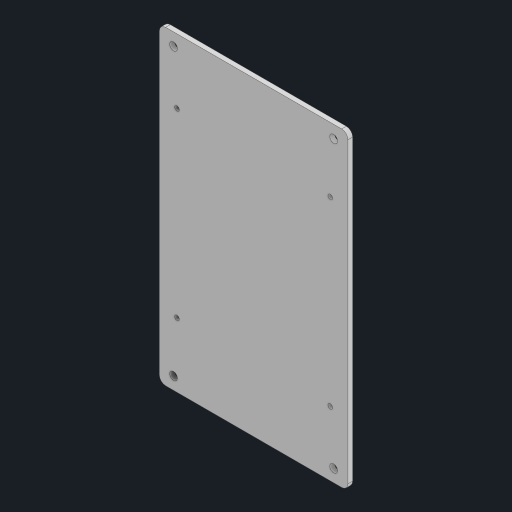
# Autodesk Inventor part: TauControllerCover
Saved by Autodesk Inventor 2023 (Build 270158000, 158)
## iProperties
Created: 2023-07-03
Part Number: TauControllerCover
Material: Generic
Document SubType Name: Sheet Metal
Designer: valer
Density: 1 g/cm^3
Sheet Metal Rule: Default
Appearance: Default
Author: valer
Autodesk Inventor part; units mm, degrees
ref_plane "YZ Plane" through (0, 0, 0) normal (1, 0, 0) x (0, 1, 0)
ref_plane "XZ Plane" through (0, 0, 0) normal (0, 1, 0) x (-1, 0, 0)
ref_plane "XY Plane" through (0, 0, 0) normal (0, 0, 1) x (1, 0, 0)
sketch "Sketch1" plane through (0, 0, 0) normal (0, 0, 1) x (1, 0, 0)
  line L0 (-28.15, 49.6305) -> (28.15, 49.6305)
  line L1 (30.15, 47.6305) -> (30.15, -47.6305)
  line L2 (28.15, -49.6305) -> (-28.15, -49.6305)
  line L3 (-30.15, -47.6305) -> (-30.15, 47.6305)
  line L4 (-30.15, 45.6305) -> (30.15, 45.6305) construction
  circle A0 centre (-25.5973, 45.6305) radius 1.25
  line L5 (0, 49.6305) -> (0, -49.6305) construction
  line L6 (-30.15, 0) -> (30.15, 0) construction
  circle A1 centre (25.5973, 45.6305) radius 1.25
  circle A2 centre (-25.5973, -45.6305) radius 1.25
  circle A3 centre (25.5973, -45.6305) radius 1.25
  arc A4 (-28.15, 49.6305) -> (-30.15, 47.6305) centre (-28.15, 47.6305) ccw
  arc A5 (30.15, 47.6305) -> (28.15, 49.6305) centre (28.15, 47.6305) ccw
  arc A6 (-30.15, -47.6305) -> (-28.15, -49.6305) centre (-28.15, -47.6305) ccw
  arc A7 (28.15, -49.6305) -> (30.15, -47.6305) centre (28.15, -47.6305) ccw
  point P0 (0, 0)
  point P1 (-30.15, 49.6305)
  point P2 (30.15, -49.6305)
  point P3 (30.15, 49.6305)
  point P4 (-30.15, -49.6305)
  point P5 (0, 0)
  dimension "d1" = 2.5
  dimension "d2" = 4
  dimension "d3" = 2
  dimension "d4" = 56.3001
  dimension "d5" = 95.2609
  dimension "d6" = 51.1946
  measures "d1" diameter of A0
  measures "d2" distance between parallel lines of L0 L4
  measures "d3" radius of A4
  measures "d4" distance of L0.start L0.end
  measures "d5" distance of L1.start L1.end
  measures "d6" distance of A1.centre A0.centre
extrude "Plate2" add sketch "Sketch1" along normal blind 1.5
sketch "Sketch2" plane through (0, 0, 1.5) normal (0, 0, 1) x (1, 0, 0)
  circle A0 centre (24.5, 29) radius 1.35
  circle A1 centre (-24.5, 29) radius 3 construction
  circle A2 centre (-24.5, 29) radius 1.35
  circle A3 centre (24.5, -29) radius 3 construction
  circle A4 centre (24.5, -29) radius 1.35
  circle A5 centre (-24.5, -29) radius 3 construction
  circle A6 centre (-24.5, -29) radius 1.35
  circle A7 centre (24.5, 29) radius 3 construction
  line L0 (-24.5, -29) -> (-24.5, 29) construction
  line L1 (-24.5, 29) -> (24.5, 29) construction
  line L2 (24.5, 29) -> (24.5, -29) construction
  line L3 (24.5, -29) -> (-24.5, -29) construction
  line L4 (-28.15, 49.6305) -> (28.15, 49.6305) projected
  line L5 (0, 49.6305) -> (0, -49.6305) construction
  line L6 (28.15, -49.6305) -> (-28.15, -49.6305) projected
  line L7 (-30.15, -47.6305) -> (-30.15, 47.6305) projected
  line L8 (-30.15, 0) -> (30.15, 0) construction
  line L9 (30.15, 47.6305) -> (30.15, -47.6305) projected
  line L10 (0, 29) -> (0, -29) construction
  line L11 (-24.5, 0) -> (24.5, 0) construction
  point P0 (0, 0)
  point P1 (0, 0)
  dimension "d9" = 6
  dimension "d10" = 2.7
  dimension "d11" = 58
  dimension "d12" = 49
  constraints: 16 end point, 10 midpoint, 8 centre point, 6 coincident, 6 equal radius, 2 parallel, 1 collinear, 1 perpendicular
  measures "d9" diameter of A5
  measures "d10" diameter of A6
  measures "d11" distance of L0.start L0.end
  measures "d12" distance of L2.end L0.start
hole "Hole1" at (-24.5, 29, 1.5) at (24.5, 29, 1.5) at (-24.5, -29, 1.5) at (24.5, -29, 1.5) direction (0, 0, -1) diameter 1.5 depth 1.5 tip angle 118
equation "\"d18\" = Thickness"
equation "\"d8\" = Thickness"
equation "\"BendRadius\" = Thickness"
equation "\"BendReliefWidth\" = Thickness"
equation "\"BendReliefDepth\" = 0.5 * Thickness"
equation "\"CornerReliefSize\" = 4 * Thickness"
equation "\"MinimumRemnant\" = 2 * Thickness"
equation "\"TransitionRadius\" = BendRadius"
equation "\"JacobiRadiusSize\" = BendRadius"
equation "\"GapSize\" = Thickness"
equation "\"Thickness\" = 1.5"
body "Solid2"
